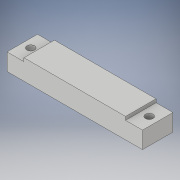
# Autodesk Inventor part: ABI_Kasten
Saved by Autodesk Inventor 2018.3 (Build 223284000, 284)
## iProperties
Created: 2019-11-22
Part Number: ABI_Kasten
Material: Generisch
Document SubType Name: Modeling
Designer: maascl
Density: 1 g/cm^3
Appearance: Vorgabe
Author: maascl
Autodesk Inventor part; units mm, degrees
ref_plane "YZ Plane" through (0, 0, 0) normal (1, 0, 0) x (0, 1, 0)
ref_plane "XZ Plane" through (0, 0, 0) normal (0, 1, 0) x (-1, 0, 0)
ref_plane "XY Plane" through (0, 0, 0) normal (0, 0, 1) x (1, 0, 0)
sketch "Skizze1" plane through (0, 0, 0) normal (0, 0, 1) x (1, 0, 0)
  line L0 (-40, -9) -> (40, -9)
  line L1 (40, -9) -> (40, 9)
  line L2 (40, 9) -> (-40, 9)
  line L3 (-40, 9) -> (-40, -9)
  line L4 (-40, -9) -> (40, 9) construction
  line L5 (40, -9) -> (-40, 9) construction
  point P0 (0, 0)
  dimension "Breite" = 80
  dimension "Höhe" = 18
  constraints: 12 end point, 2 midpoint, 2 parallel, 1 horizontal, 1 perpendicular
  measures "Breite" distance between parallel lines of L1 L3
  measures "Höhe" distance between parallel lines of L0 L2
extrude "Extrusion1" add sketch "Skizze1" along normal blind 10
sketch "Skizze2" plane through (0, 0, 10) normal (0, 0, 1) x (1, 0, 0)
  line L0 (40, 9) -> (-40, 9) projected
  line L1 (-30, -9) -> (30, -9)
  line L2 (30, -9) -> (30, 9)
  line L3 (30, 9) -> (-30, 9)
  line L4 (-30, 9) -> (-30, -9)
  line L5 (-30, -9) -> (30, 9) construction
  line L6 (30, -9) -> (-30, 9) construction
  point P0 (0, 0)
  dimension "Breite_ObererKasten" = 60
  constraints: 12 end point, 2 midpoint, 2 parallel, 1 horizontal, 1 perpendicular, 1 point on line
  measures "Breite_ObererKasten" distance between parallel lines of L2 L4
extrude "Extrusion2" add sketch "Skizze2" along normal blind 2
sketch "Skizze3" plane through (0, 0, 0) normal (0, 0, -1) x (-1, 0, 0)
  line L0 (0, -12.6) -> (0, 12.6) projected
  point P0 (0, 0)
  point P1 (-35, 0)
  point P2 (35, 0)
  dimension "Abstand_Bohrung" = 70
  constraints: 1 symmetric about line
  measures "Abstand_Bohrung" distance of point (35, 0) point (-35, 0)
hole "Bohrung1" at (35, 0, 0) at (-35, 0, 0) direction (0, 0, 1) diameter 4.5 end through all counterbore diameter 8 counterbore depth 4.6
